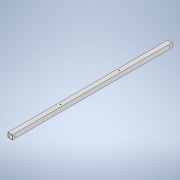
# Autodesk Inventor part: プレート保持_角柱2
Saved by Autodesk Inventor 2021 (Build 250183000, 183)
## iProperties
Created: 2022-02-03
Part Number: プレート保持_角柱2
Material: 一般
Document SubType Name: Modeling
Designer: hirohumi
Density: 1 g/cm^3
Appearance: 既定
Author: hirohumi
Autodesk Inventor part; units mm, degrees
ref_plane "YZ Plane" through (0, 0, 0) normal (1, 0, 0) x (0, 1, 0)
ref_plane "XZ Plane" through (0, 0, 0) normal (0, 1, 0) x (-1, 0, 0)
ref_plane "XY Plane" through (0, 0, 0) normal (0, 0, 1) x (1, 0, 0)
sketch "スケッチ1" plane through (0, 0, 0) normal (0, 0, 1) x (1, 0, 0)
  line L0 (7.5, 7.5) -> (-7.5, 7.5)
  line L1 (-7.5, 7.5) -> (-7.5, -7.5)
  line L2 (-7.5, -7.5) -> (7.5, -7.5)
  line L3 (7.5, -7.5) -> (7.5, 7.5)
  line L4 (7.5, 7.5) -> (-7.5, -7.5) construction
  line L5 (-7.5, 7.5) -> (7.5, -7.5) construction
  line L6 (-6.5, 6.5) -> (6.5, 6.5)
  line L7 (6.5, 6.5) -> (6.5, -6.5)
  line L8 (6.5, -6.5) -> (-6.5, -6.5)
  line L9 (-6.5, -6.5) -> (-6.5, 6.5)
  point P0 (0, 0)
  dimension "d0" = 15
  dimension "d1" = 15
  dimension "d2" = 1
  constraints: 20 end point, 4 parallel, 2 midpoint, 2 perpendicular, 1 horizontal, 3 other
  measures "d0" distance of L2.end L1.end
  measures "d1" distance of L1.end L0.end
  measures "d2" distance between parallel lines of L0 L6
extrude "押し出し1" add sketch "スケッチ1" along normal blind 540
sketch "スケッチ2" plane through (7.5, -7.5, 0) normal (1, 0, 0) x (0, 0, -1)
  circle A0 centre (-7.5, 7.5) radius 1.6
  line L0 (0, 15) -> (-540, 15) projected
  circle A1 centre (-532.5, 7.5) radius 1.6
  line L1 (-540, 0) -> (-540, 15) projected
  point P0 (0, 7.5)
  dimension "d5" = 3.2
  dimension "d6" = 7.5
  dimension "d7" = 7.5
  dimension "d8" = 3.2
  dimension "d9" = 7.5
  dimension "d10" = 7.5
  constraints: 2 centre point
  measures "d5" diameter of A0
  measures "d6" distance of point (0, 7.5) A0.centre
  measures "d7" distance from line of L0 A0.centre
  measures "d8" diameter of A1
  measures "d9" distance from line of L1 A1.centre
  measures "d10" distance from line of L0 A1.centre
extrude "押し出し2" cut sketch "スケッチ2" against normal through all
sketch "スケッチ3" plane through (-7.5, 7.5, 0) normal (0, 1, 0) x (1, 0, 0)
  circle A0 centre (7.5, -170) radius 1.6
  circle A1 centre (7.5, -370) radius 1.6
  line L0 (15, 0) -> (0, 0) projected
  point P0 (7.5, 0)
  point P1 (7.5, 0)
  dimension "d13" = 3.2
  dimension "d14" = 3.2
  dimension "d15" = 200
  dimension "d16" = 170
  constraints: 2 centre point, 2 vertical alignment, 1 midpoint
  measures "d13" diameter of A0
  measures "d14" diameter of A1
  measures "d15" distance of A1.centre A0.centre
  measures "d16" distance of A0.centre point (7.5, 0)
extrude "押し出し3" cut sketch "スケッチ3" against normal through all
